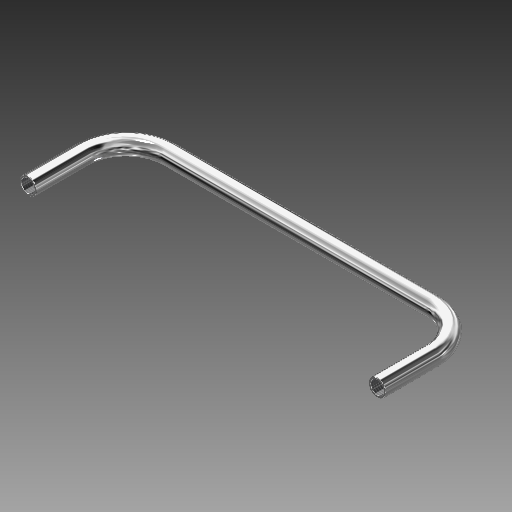
# Autodesk Inventor part: 17032101
Saved by Autodesk Inventor 2017 (Build 210142000, 142)
## iProperties
Created: 2017-03-21
Part Number: 17032101
Material: Generic
Document SubType Name: Modeling
Designer: Rendszergazda
Density: 1 g/cm^3
Appearance: Chrome - Polished
Author: Rendszergazda
Autodesk Inventor part; units mm, degrees
ref_plane "YZ Plane" through (0, 0, 0) normal (1, 0, 0) x (0, 1, 0)
ref_plane "XZ Plane" through (0, 0, 0) normal (0, 1, 0) x (-1, 0, 0)
sketch "Sketch1" plane through (0, 0, 0) normal (0, 1, 0) x (-1, 0, 0)
  line L0 (20, 0) -> (140, 0)
  line L1 (160, 20) -> (160, 45)
  line L2 (0, 45) -> (0, 20)
  arc A0 (0, 20) -> (20, 0) centre (20, 20) ccw
  arc A1 (140, 0) -> (160, 20) centre (140, 20) ccw
  point P0 (0, 0)
  point P1 (160, 0)
  dimension "d0" = 160
  dimension "d1" = 45
  dimension "d2" = 20
  constraints: 6 end point, 4 point on circle, 4 point on line, 4 tangent, 2 centre point, 1 equal radius, 1 horizontal, 1 parallel, 1 perpendicular
  measures "d0" distance of point (0, 0) point (160, 0)
  measures "d1" distance of L2.start point (0, 0)
  measures "d2" radius of A0
ref_plane "Work Plane2" through (0, 0, 45) normal (0, 0, 1) x (1, 0, 0)
sketch "Sketch2" plane through (0, 0, 45) normal (0, 0, 1) x (1, 0, 0)
  circle A0 centre (0, 0) radius 4
  circle A1 centre (0, 0) radius 3
  dimension "d4" = 8
  dimension "d5" = 6
  constraints: 2 centre point, 2 coincident
  measures "d4" diameter of A0
  measures "d5" diameter of A1
sweep "Sweep1" add profiles "Sketch2" path "Sketch1"
chamfer "Chamfer1" distance 0.2 angle 45 12 edges at (-4, 0, 45) (-4, 0, 20) (-3, 0, 45) (-20, 0, 4) (-3, 0, 20) (-140, 0, 4) (-20, 0, 3) (-156, 0, 20) (-140, 0, 3) (-156, 0, 45) (-157, 0, 20) (-157, 0, 45)
thread "Thread2"
thread "Thread3"
body "Solid1"
